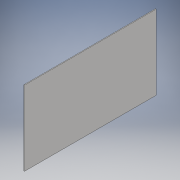
# Autodesk Inventor part: EastWall
Saved by Autodesk Inventor 2018 (Build 220112000, 112)
## iProperties
Created: 2019-04-28
Part Number: EastWall
Material: Generic
Document SubType Name: Modeling
Designer: snipe
Density: 1 g/cm^3
Appearance: Default
Author: snipe
Autodesk Inventor part; units mm, degrees
ref_plane "YZ Plane" through (0, 0, 0) normal (1, 0, 0) x (0, 1, 0)
ref_plane "XZ Plane" through (0, 0, 0) normal (0, 1, 0) x (-1, 0, 0)
ref_plane "XY Plane" through (0, 0, 0) normal (0, 0, 1) x (1, 0, 0)
sketch "Sketch1" plane through (0, 0, 0) normal (1, 0, 0) x (0, 1, 0)
  line L0 (-1295.4, 2286) -> (1295.4, 2286)
  line L1 (1295.4, 2286) -> (1295.4, -2286)
  line L2 (1295.4, -2286) -> (-1295.4, -2286)
  line L3 (-1295.4, -2286) -> (-1295.4, 2286)
  line L4 (0, 3200.4) -> (0, -3200.4) projected
  line L5 (-1813.56, 0) -> (1813.56, 0) projected
  line L6 (-1813.56, 0) -> (1813.56, 0) projected
  line L7 (0, -3200.4) -> (0, 3200.4) projected
  point P0 (0, 0)
  dimension "d0" = 2590.8
  dimension "d1" = 4572
  constraints: 8 end point, 2 parallel, 1 horizontal, 1 perpendicular, 2 other
  measures "d0" distance of L1.end L2.end
  measures "d1" distance of L0.end L1.end
extrude "Extrusion1" add sketch "Sketch1" along normal mid plane 25.4
body "Solid1"
